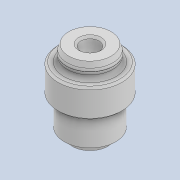
# Autodesk Inventor part: pipettetip_alignmenttool_v2
Saved by Autodesk Inventor 2021 (Build 250183000, 183)
## iProperties
Created: 2022-05-09
Part Number: pipettetip_alignmenttool_v2
Material: Generic
Document SubType Name: Modeling
Designer: to172
Density: 1 g/cm^3
Appearance: Default
Author: to172
Autodesk Inventor part; units mm, degrees
ref_plane "YZ Plane" through (0, 0, 0) normal (1, 0, 0) x (0, 1, 0)
ref_plane "XZ Plane" through (0, 0, 0) normal (0, 1, 0) x (-1, 0, 0)
ref_plane "XY Plane" through (0, 0, 0) normal (0, 0, 1) x (1, 0, 0)
sketch "Sketch1" plane through (0, 0, 0) normal (0, 0, 1) x (1, 0, 0)
  line L0 (0, 0) -> (0, 8.9988) construction
  line L1 (0, 0) -> (7.1408, 0) construction
  line L2 (0.9, 0) -> (2.3166, 18)
  line L3 (0.9, 0) -> (6.45, 0)
  line L4 (6.45, 0) -> (6.45, 7)
  line L5 (6.45, 7) -> (8, 7)
  line L6 (6.5, 18) -> (2.3166, 18)
  line L7 (6.5, 18) -> (5.85, 18)
  line L8 (5.85, 18) -> (5.85, 15)
  line L9 (5.85, 15) -> (6.5, 15)
  line L10 (6.5, 15) -> (6.5, 18)
  line L11 (5.85, 16.45) -> (5.3, 18)
  circle A0 centre (6.5, 15) radius 0.85
  line L12 (8, 7) -> (8, 14.15)
  line L13 (8, 14.15) -> (6.5, 14.15)
  line L14 (6.5, 14.15) -> (6.5, 15)
  point P0 (5.85, 15.5477)
  point P1 (6.5, 14.15)
  dimension "d0" = 7
  dimension "d1" = 6.45
  dimension "d4" = 18
  dimension "d6" = 4.5
  dimension "d7" = 0.9
  dimension "d9" = 1.7
  dimension "d10" = 3
  dimension "d11" = 0.55
  dimension "d12" = 1.55
  dimension "d18" = 6.5
  dimension "d19" = 0.65
  dimension "d20" = 8
  constraints: 30 end point, 4 perpendicular, 4 point on line, 3 horizontal, 2 parallel, 2 vertical, 1 centre point, 1 coincident, 1 tangent
  measures "d0" distance between parallel lines of L1 L5
  measures "d1" distance between parallel lines of L4 L0
  measures "d4" distance between parallel lines of L6 L1
  measures "d6" angle of L2 L0
  measures "d7" distance from line of L2.start L0
  measures "d9" diameter of A0
  measures "d10" distance between parallel lines of L6 L9
  measures "d11" distance from line of L8 L11.end
  measures "d12" distance from line of L6 L11.start
  measures "d18" distance between parallel lines of L0 L14
  measures "d19" distance between parallel lines of L10 L8
  measures "d20" distance between parallel lines of L0 L12
revolve "Revolution1" add sketch "Sketch1" angle 360 about axis through (0, 0, 0) along (0, 1, 0) contours L2 L6 L11 L8 A0 L13 L12 L5 L4 L3
chamfer "Chamfer1" distance 0.5 angle 45 3 edges at (-8, 7, 0) (-2.3166, 18, 0) (-8, 14.15, 0)
fillet "Fillet1" radius 2 2 edges at (-5.85, 15.5477, 0) (-5.85, 16.45, 0)
sketch "Sketch2" plane through (0, 0, 0) normal (0, -1, 0) x (1, 0, 0)
  circle A0 centre (0, 0) radius 6.45 projected
  circle A1 centre (0, 0) radius 0.9 projected
extrude "Extrusion1" add sketch "Sketch2" along normal blind 2
chamfer "Chamfer2" distance 2 angle 45 2 edges at (-0.9, -2, 0) (-6.45, -2, 0)
body "Solid1"
